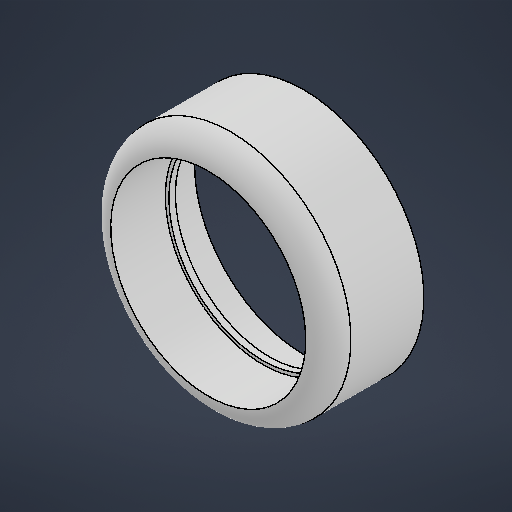
# Autodesk Inventor part: Forward_Coupler
Saved by Autodesk Inventor 2026.1 (Build 301233000, 233)
## iProperties
Created: 2025-11-13
Part Number: Forward_Coupler
Material: Generic
Document SubType Name: Modeling
Designer: 1char
Mass: 110.414 g
Surface Area: 336.712 cm^2
Volume: 110.414 cm^3
Density: 1 g/cm^3
Appearance: Default
Author: 1char
Autodesk Inventor part; units mm, degrees
ref_plane "YZ Plane" through (0, 0, 0) normal (1, 0, 0) x (0, 1, 0)
ref_plane "XZ Plane" through (0, 0, 0) normal (0, 1, 0) x (-1, 0, 0)
ref_plane "XY Plane" through (0, 0, 0) normal (0, 0, 1) x (1, 0, 0)
sketch "Sketch5" plane through (0, 0, 0) normal (1, 0, 0) x (0, 1, 0)
  line L0 (0, 0) -> (-118.6879, 0) construction
  line L1 (-28.75, 44.65) -> (-3.75, 44.65)
  arc A0 (-18.4, 55) -> (-28.75, 44.65) centre (-18.4, 44.65) ccw
  line L2 (-18.4, 55) -> (15, 55)
  line L3 (-0.75, 43.05) -> (-0.75, 50)
  line L4 (-0.75, 50) -> (15, 50)
  line L5 (15, 50) -> (15, 55)
  line L6 (-3.75, 44.65) -> (-3.75, 43.05)
  line L7 (-3.75, 43.05) -> (-0.75, 43.05)
  dimension "d14" = 89.3
  dimension "d15" = 0.75
  dimension "d16" = 1.6
  dimension "d17" = 3
  dimension "d18" = 15
  dimension "d19" = 5
  dimension "d20" = 100
  dimension "d21" = 25
  constraints: 16 end point, 3 horizontal, 3 perpendicular, 2 point on circle, 2 vertical, 1 centre point, 1 point on line, 1 tangent
  measures "d14" diameter of L1 L0
  measures "d15" horizontal distance of L3.start L0.start
  measures "d16" distance between parallel lines of L1 L7
  measures "d17" distance of L6.end L3.start
  measures "d18" distance from line of L5 L0.start
  measures "d19" distance between parallel lines of L4 L2
  measures "d20" diameter of L4 L0
  measures "d21" distance of L1.start L1.end
revolve "Revolution1" add sketch "Sketch5" angle 360 about axis through (0, 0, 0) along (0, -1, 0)
body "Solid3"
